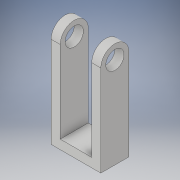
# Autodesk Inventor part: CollectorHolder
Saved by Autodesk Inventor 2017 (Build 210142000, 142)
## iProperties
Created: 2017-04-19
Part Number: CollectorHolder
Material: Generic
Document SubType Name: Modeling
Designer: User
Density: 1 g/cm^3
Appearance: Default
Mass: 12.4911 g
Surface Area: 60.7785 cm^2
Volume: 12.4911 cm^3
Author: User
Autodesk Inventor part; units mm, degrees
ref_plane "YZ Plane" through (0, 0, 0) normal (1, 0, 0) x (0, 1, 0)
ref_plane "XZ Plane" through (0, 0, 0) normal (0, 1, 0) x (-1, 0, 0)
ref_plane "XY Plane" through (0, 0, 0) normal (0, 0, 1) x (1, 0, 0)
sketch "Sketch1" plane through (0, 0, 0) normal (1, 0, 0) x (0, 1, 0)
  circle A0 centre (0, 0) radius 6.35
  arc A1 (0, -9.779) -> (0, 9.779) centre (0, 0) ccw
  line L0 (0, 9.779) -> (-63.5, 9.779)
  line L1 (-63.5, 9.779) -> (-63.5, -9.779)
  line L2 (-63.5, -9.779) -> (0, -9.779)
  dimension "d0" = 12.7
  dimension "d1" = 19.558
  dimension "d2" = 63.5
  dimension "d3" = 19.558
  constraints: 6 end point, 2 centre point, 2 coincident, 2 perpendicular, 2 point on circle, 1 horizontal, 1 tangent
  measures "d0" diameter of A0
  measures "d1" diameter of A1
  measures "d2" distance of L0.start L0.end
  measures "d3" distance of L0.end L1.end
extrude "Extrusion1" add sketch "Sketch1" along normal blind 34.671
sketch "Sketch2" plane through (0, -63.5, 9.779) normal (0, 0, 1) x (1, 0, 0)
  line L0 (34.671, 63.5) -> (34.671, 0) projected
  line L1 (0, 0) -> (0, 63.5) projected
  line L2 (0, 73.279) -> (34.671, 73.279) projected
  line L3 (0, 0) -> (34.671, 0) projected
  line L4 (6.35, 73.279) -> (28.321, 73.279)
  line L5 (28.321, 73.279) -> (28.321, 6.35)
  line L6 (28.321, 6.35) -> (6.35, 6.35)
  line L7 (6.35, 6.35) -> (6.35, 73.279)
  dimension "d8" = 6.35
  dimension "d12" = 6.35
  dimension "d13" = 6.35
  constraints: 8 end point, 2 parallel, 1 horizontal, 1 perpendicular, 1 point on line
  measures "d8" distance between parallel lines of L1 L7
  measures "d12" distance between parallel lines of L0 L5
  measures "d13" distance between parallel lines of L3 L6
extrude "Extrusion2" cut sketch "Sketch2" against normal blind 32.004
body "Solid1"
